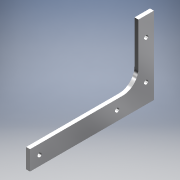
# Autodesk Inventor part: Back brace 2
Saved by Autodesk Inventor 2019.4 (Build 234330000, 330)
## iProperties
Created: 2020-01-06
Part Number: Back brace 2
Material: Aluminum 6061
Document SubType Name: Modeling
Designer: Mark
Mass: 54 g
Surface Area: 98.5 cm^2
Volume: 20 cm^3
Density: 2.7 g/cm^3
Appearance: Aluminum - Flat
Author: Mark
Autodesk Inventor part; units mm, degrees
ref_plane "YZ Plane" through (0, 0, 0) normal (1, 0, 0) x (0, 1, 0)
ref_plane "XZ Plane" through (0, 0, 0) normal (0, 1, 0) x (-1, 0, 0)
ref_plane "XY Plane" through (0, 0, 0) normal (0, 0, 1) x (1, 0, 0)
sketch "Sketch1" plane through (0, 0, 0) normal (1, 0, 0) x (0, 1, 0)
  line L0 (0, 0) -> (25, 0)
  line L1 (25, 0) -> (25, -160)
  line L2 (25, -160) -> (0, -160)
  line L3 (0, -160) -> (0, 0)
  line L4 (25, -160) -> (100, -160)
  line L5 (100, -160) -> (100, -140)
  line L6 (100, -140) -> (25, -140)
  line L7 (25, -140) -> (25, -160)
  dimension "d0" = 25
  dimension "d1" = 160
  dimension "d2" = 75
  dimension "d3" = 20
  constraints: 16 end point, 4 parallel, 2 horizontal, 2 perpendicular
  measures "d0" distance of L1.end L2.end
  measures "d1" distance of L0.end L1.end
  measures "d2" distance of L6.end L5.end
  measures "d3" distance of L4.end L5.end
extrude "Extrusion1" add sketch "Sketch1" along normal blind 5
sketch "Sketch2" plane through (0, 26.1364, -99.0909) normal (-1, 0, 0) x (0, 0, 1)
  circle A0 centre (-13.4091, -13.6364) radius 2.75
  line L0 (-60.9091, 50) -> (-60.9091, -26.1364)
  line L1 (-60.9091, -26.1364) -> (80, -26.1364)
  circle A1 centre (-50.9091, -1.1364) radius 2.75
  circle A2 centre (-50.9091, 48.8636) radius 2.75
  circle A3 centre (86.5909, -13.6364) radius 2.75
  line L2 (-60.9091, 73.8636) -> (-60.9091, -26.1364) projected
  line L3 (-60.9091, -26.1364) -> (99.0909, -26.1364) projected
  point P0 (0, 0)
  dimension "d15" = 5.5
  dimension "d17" = 47.5
  dimension "d16" = 12.5
  dimension "d12" = 5.5
  dimension "d14" = 10
  dimension "d13" = 25
  dimension "d9" = 5.5
  dimension "d11" = 10
  dimension "d10" = 50
  dimension "d6" = 5.5
  dimension "d8" = 100
  dimension "d7" = 12.5
  constraints: 4 centre point, 4 end point, 2 collinear
  measures "d15" diameter of A0
  measures "d17" distance from line of L0 A0.centre
  measures "d16" distance from line of L1 A0.centre
  measures "d12" diameter of A1
  measures "d14" distance from line of L0 A1.centre
  measures "d13" distance from line of L1 A1.centre
  measures "d9" diameter of A2
  measures "d11" distance from line of A2.centre L0
  measures "d10" distance of A1.centre A2.centre
  measures "d6" diameter of A3
  measures "d8" distance of A0.centre A3.centre
  measures "d7" distance from line of L1 A3.centre
extrude "Extrusion2" cut sketch "Sketch2" against normal blind 5
fillet "Fillet1" radius 20 1 edges at (2.5, 25, -140)
body "Solid1"
